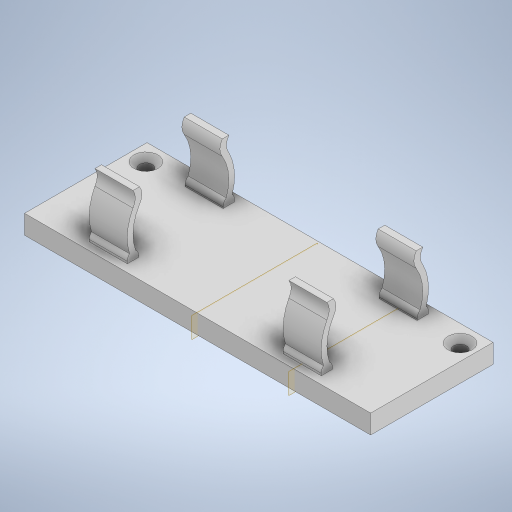
# Autodesk Inventor part: powerbank_mount
Saved by Autodesk Inventor 2024 (Build 280153000, 153)
## iProperties
Created: 2024-02-01
Part Number: powerbank_mount
Material: Generic
Document SubType Name: Modeling
Designer: crow
Density: 1 g/cm^3
Appearance: Default
Author: crow
Autodesk Inventor part; units mm, degrees
ref_plane "YZ Plane" through (0, 0, 0) normal (1, 0, 0) x (0, 1, 0)
ref_plane "XZ Plane" through (0, 0, 0) normal (0, 1, 0) x (-1, 0, 0)
ref_plane "XY Plane" through (0, 0, 0) normal (0, 0, 1) x (1, 0, 0)
sketch "Sketch1" plane through (0, 0, 0) normal (0, 1, 0) x (-1, 0, 0)
  line L0 (41.305, -11.6) -> (-41.305, -11.6) construction
  line L1 (0, 107.889) -> (0, -128.889) construction
  line L2 (45.5, -16.1) -> (-45.5, -16.1)
  line L3 (-45.5, -16.1) -> (-45.5, 16.1)
  line L4 (-45.5, 16.1) -> (45.5, 16.1)
  line L5 (45.5, 16.1) -> (45.5, -16.1)
  line L6 (62.4324, 0) -> (-80.3334, 0) construction
  point P0 (0, 0)
  point P1 (45.5, 0)
  point P2 (0, 16.1)
  point P3 (0, -11.6)
  dimension "d1" = 82.61
  dimension "d2" = 91
  dimension "d3" = 32.2
  dimension "d4" = 4.5
  constraints: 14 end point, 4 horizontal, 3 midpoint, 3 point on line, 2 coincident, 2 parallel, 2 vertical, 1 perpendicular
  measures "d1" distance of L0.start L0.end
  measures "d2" distance of L3.end L4.end
  measures "d3" distance of L2.end L3.end
  measures "d4" distance from line of L2 L0.start
extrude "Extrusion1" add sketch "Sketch1" along normal blind 5
sketch "Sketch2" plane through (0, 5, 0) normal (0, 1, 0) x (1, 0, 0)
  line L0 (-45.5, -16.1) -> (45.5, -16.1) projected
  line L1 (45.5, -16.1) -> (45.5, 16.1) projected
  line L2 (45.5, 16.1) -> (-45.5, 16.1) projected
  line L3 (-45.5, 16.1) -> (-45.5, -16.1) projected
  point P0 (0, 0)
  point P1 (41.305, 11.6)
  point P2 (-41.305, 11.6)
  point P3 (41.305, 11.6)
  point P4 (-41.305, 11.6)
  constraints: 2 coincident
hole "Hole1" at (41.305, 5, -11.6) at (-41.305, 5, -11.6) direction (0, -1, 0) diameter 3.4 depth 5 countersink diameter 6.3 countersink angle 90 clearance for "Countersunk Flat Head Screw ISO 2009/7046" size "M3" standard "ISO"
ref_plane "Work Plane1" through (25.5, 0, 16.1) normal (1, 0, 0) x (0, 0, -1)
ref_plane "Work Plane2" through (0, 0, 16.1) normal (1, 0, 0) x (0, 0, -1)
sketch "Sketch3" plane through (25.5, 0, 16.1) normal (1, 0, 0) x (0, 0, -1)
  line L0 (0, 5) -> (32.2, 5) projected
  line L1 (2, 5) -> (5, 5)
  line L2 (5, 5) -> (5, 7)
  line L3 (5, 7) -> (4.18, 7)
  line L4 (2, 7) -> (2, 5)
  line L5 (16.1, 17.288) -> (16.1, -5.2059) construction
  line L6 (0, 0) -> (0, 5) construction
  arc A0 (3.4943, 16.9472) -> (3.4943, 20.9472) centre (0.622, 18.9472) ccw
  arc A1 (5.2405, 16.979) -> (5.2223, 20.9472) centre (2.3482, 18.9499) ccw
  line L7 (3.4943, 20.9472) -> (5.2223, 20.9472)
  arc A2 (3.4943, 16.9472) -> (2.5975, 7) centre (15, 10.896) ccw
  arc A3 (5.2405, 16.979) -> (4.18, 7) centre (15, 10.896) ccw
  line L8 (2.5975, 7) -> (2, 7)
  line L9 (27.2, 5) -> (27.2, 7)
  line L10 (27.2, 7) -> (28.02, 7)
  line L11 (30.2, 7) -> (30.2, 5)
  line L12 (28.7057, 5) -> (28.7057, 18.917) construction
  arc A4 (28.7057, 20.9472) -> (28.7057, 16.9472) centre (31.578, 18.9472) ccw
  arc A5 (26.9777, 20.9472) -> (26.9595, 16.979) centre (29.8518, 18.9499) ccw
  line L13 (28.7057, 20.9472) -> (26.9777, 20.9472)
  arc A6 (29.6025, 7) -> (28.7057, 16.9472) centre (17.2, 10.896) ccw
  arc A7 (28.02, 7) -> (26.9595, 16.979) centre (17.2, 10.896) ccw
  line L14 (29.6025, 7) -> (30.2, 7)
  point P0 (16.1, 0)
  dimension "d20" = 3
  dimension "d21" = 2
  dimension "d23" = 2
  dimension "d25" = 4
  dimension "d26" = 3.5
  dimension "d27" = 3.5
  dimension "d31" = 16.1
  dimension "d32" = 1.5
  dimension "d33" = 0.5975
  dimension "d34" = 13
  constraints: 26 end point, 16 point on circle, 13 symmetric about line, 8 centre point, 3 parallel, 3 point on line, 2 horizontal, 1 perpendicular, 1 vertical, 4 other
  measures "d20" distance of L2.end L4.start
  measures "d21" distance of L1.end L2.end
  measures "d23" distance between parallel lines of L6 L4
  measures "d25" distance of A0.start L7.start
  measures "d26" radius of A0
  measures "d27" radius of A1
  measures "d31" distance between parallel lines of L5 L6
  measures "d32" radial gap between concentric circles of A3 A2
  measures "d33" distance of L8.start L4.start
  measures "d34" radius of A2
extrude "Extrusion2" add sketch "Sketch3" along normal mid plane 10
mirror "Mirror1" about plane through (0, 0, 16.1) normal (1, 0, 0) of "Extrusion2"
fillet "Fillet1" radius 2 8 edges at (25.5, 7, 14.1) (25.5, 7, 11.1) (-25.5, 7, 14.1) (-25.5, 7, 11.1) (25.5, 7, -11.1) (25.5, 7, -14.1) (-25.5, 7, -14.1) (-25.5, 7, -11.1)
body "Solid1"
